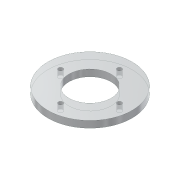
# Autodesk Inventor part: M20 - Flange Connector
Saved by Autodesk Inventor 2016 (Build 200138000, 138)
## iProperties
Created: 2017-03-02
Part Number: M20 - Flange Connector
Material: ABS Plastic
Document SubType Name: Modeling
Designer: Fernando
Stock Number: 0
Mass: 49.1112 g
Surface Area: 160.118 cm^2
Volume: 46.3313 cm^3
Density: 1.06 g/cm^3
Appearance: Clear
SurfaceArea_m2: .02
Author: Fernando
Autodesk Inventor part; units mm, degrees
ref_plane "YZ Plane" through (0, 0, 0) normal (1, 0, 0) x (0, 1, 0)
ref_plane "XZ Plane" through (0, 0, 0) normal (0, 1, 0) x (-1, 0, 0)
ref_plane "XY Plane" through (0, 0, 0) normal (0, 0, 1) x (1, 0, 0)
sketch "Sketch2" plane through (0, 0, 0) normal (0, 0, 1) x (1, 0, 0)
  circle A0 centre (0, 0) radius 25
  circle A1 centre (0, 0) radius 50
  dimension "d11" = 100
  dimension "d12" = 50
  constraints: 2 centre point, 2 coincident
  measures "d11" diameter of A1
  measures "d12" diameter of A0
extrude "Extrusion2" add sketch "Sketch2" along normal blind 8
sketch "Sketch3" plane through (0, 0, 8) normal (0, 0, 1) x (1, 0, 0)
  point P0 (0, 0)
  point P1 (35, 0)
  dimension "d15" = 35
  constraints: 1 horizontal alignment
  measures "d15" distance of point (0, 0) point (35, 0)
hole "Hole1" at (35, 0, 8) direction (0, 0, -1) diameter 4.5 depth 8 tip angle 118
pattern_circular "Circular Pattern1" count 4 over 360 about axis through (0, 0, 0) along (0, 0, 1) of "Hole1"
sketch "Sketch4" plane through (0, 0, 0) normal (0, 0, -1) x (-1, 0, 0)
  line L0 (0, 0) -> (28.2843, 28.2843)
  line L1 (0, 0) -> (17.6035, 0)
  dimension "d26" = 45
  dimension "d27" = 40
  constraints: 4 end point, 1 horizontal
  measures "d26" angle of L0 L1
  measures "d27" distance of L0.start L0.end
hole "Hole2" at (-28.2843, 28.2843, 0) direction (0, 0, 1) diameter 4.2 depth 8 tip angle 118 countersink diameter 8 countersink angle 90
pattern_circular "Circular Pattern2" count 2 over 360 about axis through (0, 0, 0) along (0, 0, 1) of "Hole2"
body "Solid2"
